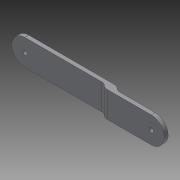
# Autodesk Inventor part: ramie3
Saved by Autodesk Inventor 2013 (Build 170138000, 138)
## iProperties
Created: 2013-03-06
Part Number: ramie3
Material: Generic
Document SubType Name: Modeling
Designer: Masta
Density: 1 g/cm^3
Author: Masta
Autodesk Inventor part; units mm, degrees
ref_plane "YZ Plane" through (0, 0, 0) normal (1, 0, 0) x (0, 1, 0)
ref_plane "XZ Plane" through (0, 0, 0) normal (0, 1, 0) x (-1, 0, 0)
ref_plane "XY Plane" through (0, 0, 0) normal (0, 0, 1) x (1, 0, 0)
sketch "Sketch1" plane through (0, 0, 0) normal (0, 1, 0) x (-1, 0, 0)
  line L0 (-50, 10) -> (-18.2962, 10)
  line L1 (-50, -10) -> (-18.2962, -10)
  arc A0 (50, -10) -> (50, 10) centre (50, 0) ccw
  arc A1 (-50, 10) -> (-50, -10) centre (-50, 0) ccw
  circle A2 centre (50, 0) radius 1.6
  line L2 (0, 0) -> (0, -27.365) construction
  line L3 (0, 0) -> (19.8022, 0) construction
  circle A3 centre (50, 0) radius 4.75
  circle A4 centre (-50, 0) radius 1.6
  circle A5 centre (-50, 0) radius 4.75
  line L4 (-13.5485, -10) -> (-13.5485, 10)
  line L5 (-18.2962, -10) -> (-18.2962, 10)
  line L6 (-18.2962, 10) -> (-13.5485, 10)
  line L7 (-13.5485, 10) -> (50, 10)
  line L8 (-18.2962, -10) -> (-13.5485, -10)
  line L9 (-13.5485, -10) -> (50, -10)
  dimension "d1" = 100
  dimension "d2" = 10
  dimension "d3" = 3.2
  dimension "d4" = 9.5
  constraints: 20 end point, 10 perpendicular, 9 parallel, 9 tangent, 6 centre point, 4 coincident, 4 point on circle, 3 horizontal, 3 symmetric about line, 2 point on line, 3 other
  measures "d1" distance of L0.start L7.end
  measures "d2" radius of A1
  measures "d3" diameter of A2
  measures "d4" diameter of A3
extrude "Extrusion1" add sketch "Sketch1" against normal blind 3 contours L0 L5 L1 A1 | L6 L4 L8 L5 | A5
extrude "Extrusion2" cut sketch "Sketch1" against normal blind 0.3 contours A3 | A5
extrude "Extrusion3" add sketch "Sketch1" along normal blind 3 contours L6 L4 L8 L5 | L7 A0 L9 L4 | A3
fillet "Fillet1" radius 5 4 edges at (18.2962, 3, 0) (18.2962, 0, 0) (13.5485, 0, 0) (13.5485, -3, 0)
body "Solid1"
